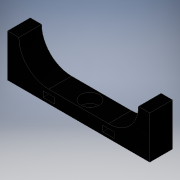
# Autodesk Inventor part: CT_Holder
Saved by Autodesk Inventor 2016 (Build 200138000, 138)
## iProperties
Created: 2018-04-30
Part Number: CT_Holder
Material: Generic
Document SubType Name: Modeling
Designer: Phil Erle
Density: 1 g/cm^3
Appearance: Black
Author: Phil Erle
Autodesk Inventor part; units mm, degrees
ref_plane "YZ Plane" through (0, 0, 0) normal (1, 0, 0) x (0, 1, 0)
ref_plane "XZ Plane" through (0, 0, 0) normal (0, 1, 0) x (-1, 0, 0)
ref_plane "XY Plane" through (0, 0, 0) normal (0, 0, 1) x (1, 0, 0)
sketch "Sketch1" plane through (0, 0, 0) normal (0, 0, 1) x (1, 0, 0)
  line L0 (-25, -4) -> (25, -4)
  line L1 (25, -4) -> (25, 4)
  line L2 (25, 4) -> (-25, 4)
  line L3 (-25, 4) -> (-25, -4)
  line L4 (-25, -4) -> (25, 4) construction
  line L5 (25, -4) -> (-25, 4) construction
  point P0 (0, 0)
  dimension "d0" = 50
  dimension "d1" = 8
  constraints: 12 end point, 2 midpoint, 2 parallel, 1 horizontal, 1 perpendicular
  measures "d0" distance of L1.end L2.end
  measures "d1" distance of L0.end L1.end
extrude "Extrusion1" add sketch "Sketch1" along normal blind 15
sketch "Sketch2" plane through (-25, 4, 0) normal (0, 1, 0) x (1, 0, 0)
  circle A0 centre (35.5, -15) radius 10.5
  circle A1 centre (14.5, -15) radius 10.5
  line L0 (35.5, -15) -> (14.5, -15) construction
  line L1 (50, 0) -> (0, 0) construction
  line L2 (35.5, -4.5) -> (14.5, -4.5)
  line L3 (35.5, -4.5) -> (25, -15)
  line L4 (25, -15) -> (14.5, -4.5)
  point P0 (25, 0)
  point P1 (25, -15)
  point P2 (25, 0)
  point P3 (25, 0)
  dimension "d4" = 21
  dimension "d5" = 21
  dimension "d6" = 21
  constraints: 8 end point, 4 vertical alignment, 3 midpoint, 1 horizontal, 4 other
  measures "d6" distance of L0.start L0.end
extrude "Extrusion2" cut sketch "Sketch2" against normal blind 15
sketch "Sketch3" plane through (-25, -4, 0) normal (0, -1, 0) x (1, 0, 0)
  line L0 (12.5, 1) -> (16.5, 1)
  line L1 (16.5, 1) -> (16.5, 3)
  line L2 (16.5, 3) -> (12.5, 3)
  line L3 (12.5, 3) -> (12.5, 1)
  line L4 (37.5, 1) -> (33.5, 1)
  line L5 (33.5, 1) -> (33.5, 3)
  line L6 (33.5, 3) -> (37.5, 3)
  line L7 (37.5, 3) -> (37.5, 1)
  line L8 (0, 0) -> (50, 0) projected
  point P0 (25, 0)
  point P1 (14.5, 3)
  point P2 (14.5, 4.5)
  point P3 (35.5, 4.5)
  point P4 (35.5, 3)
  dimension "d9" = 2
  dimension "d10" = 4
  dimension "d11" = 4
  dimension "d12" = 1
  constraints: 16 end point, 4 parallel, 2 horizontal, 2 midpoint, 2 perpendicular, 2 point on line, 2 vertical alignment
  measures "d9" distance of L2.end L0.start
  measures "d10" distance of L0.start L0.end
  measures "d11" distance of L4.start L4.end
  measures "d12" distance between parallel lines of L8 L0
extrude "Extrusion3" cut sketch "Sketch3" against normal blind 15
sketch "Sketch4" plane through (-10.5, 4, 4.5) normal (0, 0, 1) x (1, 0, 0)
  point P0 (10.5, -4)
  point P1 (10.5, -4)
  constraints: 1 coincident
hole "Hole1" at (0, 0, 4.5) direction (0, 0, -1) diameter 3.4 depth 8 tip angle 118 counterbore diameter 6.5 counterbore depth 3.4 clearance for "Socket Head Cap Screw DIN EN ISO 4762" size "M3" standard "DIN"
body "Solid1"
